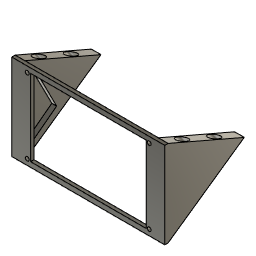
Display_Stand v2 (Autodesk Fusion 360 design; units mm, degrees)
Autodesk Fusion 360 part; units mm, degrees
sketch "Sketch2" plane through (0, 0, 0) normal (0, 1, 0) x (1, 0, 0)
  line L0 (0, 0) -> (126, 0) construction
  line L1 (0, 0) -> (0, -77) construction
  circle A0 centre (126, 0) radius 2
  circle A1 centre (0, 0) radius 2
  circle A2 centre (0, -77) radius 2
  line L2 (126, 0) -> (126, -77) construction
  circle A3 centre (126, -77) radius 2
  line L3 (3.4555, -78.0942) -> (122.9555, -78.0942)
  line L4 (122.9555, -78.0942) -> (122.9555, 0.9058)
  line L5 (122.9555, 0.9058) -> (3.4555, 0.9058)
  line L6 (3.4555, 0.9058) -> (3.4555, -78.0942)
  line L7 (-6, -77) -> (-6, -83) construction
  line L8 (-6, -83) -> (0, -83) construction
  line L9 (-6, -83) -> (132, -83)
  line L10 (132, -83) -> (132, 6)
  line L11 (132, 6) -> (-6, 6)
  line L12 (-6, 6) -> (-6, -83)
  dimension "d16" = 4
  dimension "d17" = 4
  dimension "d18" = 4
  dimension "d20" = 4
  dimension "d23" = 6
  dimension "d24" = 6
  dimension "d25" = 138
  dimension "d26" = 89
  constraint coincident L0.start L1.start
  constraint horizontal L0
  constraint perpendicular L0 L1
  constraint coincident L0.end A0.centre
  constraint coincident L1.end A2.centre
  constraint vertical L2
  constraint coincident L2.end A3.centre
  constraint horizontal L3
  constraint vertical L4
  constraint horizontal L5
  constraint vertical L6
  constraint vertical L7
  constraint horizontal L8
  constraint horizontal L9
  constraint vertical L10
  constraint horizontal L11
  constraint vertical L12
  measures "d16" diameter of A0
  measures "d17" diameter of A1
  measures "d18" diameter of A2
  measures "d20" diameter of A3
  measures "d23" distance of L1.end L7.start
  measures "d24" distance of L1.end L8.end
  measures "d25" distance of L7.end L9.end
  measures "d26" distance of L7.end L11.end
extrude "Extrude2" add sketch "Sketch2" against normal blind 3.5
sketch "Sketch3" plane through (132, 0, 0) normal (1, 0, 0) x (0, 1, 0)
  line L0 (0, -6) -> (0, 83)
  line L1 (0, 83) -> (-3.5, 83)
  line L2 (-3.5, 83) -> (-3.5, -6)
  line L3 (-3.5, -6) -> (0, -6)
  line L4 (0, -6) -> (78.6469, 49.0692)
  line L5 (0, -6) -> (96.0102, -6) construction
  line L6 (78.6469, 49.0692) -> (0, 83)
  dimension "d29" = 35
  constraint horizontal L5
  constraint coincident L0.start L3.end
  constraint coincident L0.end L1.start
  measures "d29" angle of L4 L5
extrude "Extrude3" add sketch "Sketch3" along normal blind 10
sketch "Sketch4" plane through (-6, 0, 0) normal (-1, 0, 0) x (0, -1, 0)
  line L0 (0, 83) -> (0, -6)
  line L1 (0, -6) -> (3.5, -6)
  line L2 (3.5, -6) -> (3.5, 83)
  line L3 (3.5, 83) -> (0, 83)
  line L4 (0, 83) -> (-78.6469, 49.0692)
  line L5 (-78.6469, 49.0692) -> (0, -6)
  point P0 (-78.6469, 49.0692)
  constraint coincident L0.start L3.end
  constraint coincident P0 L4.end
  constraint coincident L0.end L1.start
extrude "Extrude4" add sketch "Sketch4" along normal blind 10
sketch "Sketch5" plane through (0, 2.8191, -4.0261) normal (0, 0.573576, -0.819152) x (-1, 0, 0)
  line L0 (-132, -3.4415) -> (-132, 92.5687)
  line L1 (-132, 92.5687) -> (-142, 92.5687)
  line L2 (-142, 92.5687) -> (-142, -3.4415)
  line L3 (-142, -3.4415) -> (-132, -3.4415)
  line L4 (-137, 92.5687) -> (-137, -3.4415) construction
  line L5 (6, 47.6068) -> (-132, 47.6068)
  line L6 (-63, 47.6068) -> (-63, 87.5387) construction
  line L7 (-137, 92.5687) -> (-137, 77.5687) construction
  circle A0 centre (-137, 77.5687) radius 2
  circle A1 centre (-137, 58.7979) radius 2
  circle A2 centre (11, 77.5687) radius 2
  circle A3 centre (11, 58.7979) radius 2
  circle A4 centre (-137, 77.5687) radius 4
  circle A5 centre (-137, 58.7979) radius 4
  circle A6 centre (11, 58.7979) radius 4
  circle A7 centre (11, 77.5687) radius 4
  dimension "d34" = 15
  dimension "d35" = 4
  dimension "d36" = 4
  dimension "d39" = 8
  dimension "d40" = 8
  constraint midpoint L1 L4.start
  constraint midpoint L3 L4.end
  constraint midpoint L5 L6.start
  constraint perpendicular L3 L6
  constraint perpendicular L1 L7
  constraint coincident L7.end A0.centre
  constraint coincident L4 A1.centre
  constraint symmetric L6 A0 A2
  constraint symmetric L6 A1 A3
  constraint concentric A1 A5
  constraint symmetric L6 A4 A7
  constraint symmetric L6 A5 A6
  measures "d34" distance of L4.start L7.end
  measures "d35" diameter of A0
  measures "d36" diameter of A1
  measures "d39" diameter of A4
  measures "d40" diameter of A5
extrude "Extrude6" cut sketch "Sketch5" against normal blind 64 contours A0 | A1 | A2 | A3
ref_plane "WorkPlane1" through (137, 37.0292, 24.8112) normal (0, 0.573576, -0.819152) x (0, 0.819152, 0.573576)
sketch "Sketch6" plane through (137, 37.0292, 24.8112) normal (0, 0.573576, -0.819152) x (0, 0.819152, 0.573576)
  circle A0 centre (33.0958, 0) radius 4
  circle A1 centre (14.1568, -0.0063) radius 4
  line L0 (3.0432, -143) -> (3.0432, -5)
  line L1 (3.0432, -74) -> (11.3701, -74) construction
  circle A2 centre (33.0958, -148) radius 4
  circle A3 centre (14.1568, -147.9937) radius 4
  dimension "d44" = 8
  dimension "d45" = 8
  constraint midpoint L0 L1.start
  constraint perpendicular L0 L1
  constraint symmetric A0 L1 A2
  constraint symmetric A1 L1 A3
  measures "d44" diameter of A0
  measures "d45" diameter of A1
extrude "Extrude7" cut sketch "Sketch6" against normal blind 65
sketch "Sketch7" plane through (-6, 0, 0) normal (1, 0, 0) x (0, 1, 0)
  line L0 (0, 83) -> (0, -6)
  line L1 (0, -6) -> (78.6469, 49.0692)
  line L2 (78.6469, 49.0692) -> (0, 83)
  line L3 (2.5489, 73.8327) -> (2.5489, 2.9392)
  line L4 (2.5489, 2.9392) -> (32.8483, 25.9556)
  line L5 (32.8483, 25.9556) -> (10.651, 69.2676)
  line L6 (10.651, 69.2676) -> (2.5489, 73.8327)
  constraint vertical L3
extrude "Extrude8" cut sketch "Sketch7" against normal blind 5 contours L3 L4 L5 L6
